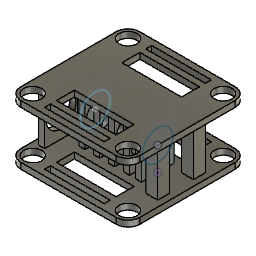
ROV frame sketch v1 (Autodesk Fusion 360 design; units mm, degrees)
Autodesk Fusion 360 part; units mm, degrees
sketch "Sketch3" plane through (0, 0, 0) normal (0, 0, 1) x (1, 0, 0)
  line L0 (80, 100) -> (-80, 100)
  line L1 (-100, 80) -> (-100, -80)
  line L2 (-80, -100) -> (80, -100)
  line L3 (100, -80) -> (100, 80)
  line L4 (100, 100) -> (-94.1421, -94.1421) construction
  line L5 (-100, 100) -> (100, -100) construction
  circle A0 centre (80, -80) radius 15
  circle A1 centre (80, 80) radius 15
  circle A2 centre (-80, -80) radius 15
  line L6 (-90, -5) -> (-90, -60)
  line L7 (-90, -60) -> (-80, -60)
  line L8 (-80, -60) -> (-80, -5)
  line L9 (-80, 45.4617) -> (-80, 5)
  line L10 (-80, 5) -> (-80, 60)
  line L11 (-80, 60) -> (-90, 60)
  line L12 (-90, 60) -> (-90, 5)
  line L13 (-90, -5) -> (-80, -5)
  line L14 (-80, 5) -> (-90, 5)
  arc A3 (100, 80) -> (80, 100) centre (80, 80) ccw
  arc A4 (80, -100) -> (100, -80) centre (80, -80) ccw
  arc A5 (-100, -80) -> (-80, -100) centre (-80, -80) ccw
  arc A6 (-80, 100) -> (-100, 80) centre (-80, 80) ccw
  line L15 (-50, 90) -> (50, 90)
  line L16 (50, 90) -> (50, 80)
  line L17 (50, 80) -> (-50, 80)
  line L18 (-50, 80) -> (-50, 90)
  line L19 (-50, -80) -> (50, -80)
  line L20 (50, -80) -> (50, -90)
  line L21 (50, -90) -> (-50, -90)
  line L22 (-50, -90) -> (-50, -80)
  line L23 (-80, -5) -> (-80, -60)
  line L24 (-80, 5) -> (-80, 60)
  circle A7 centre (-80, 80) radius 15
  line L25 (70, -20) -> (90, -20)
  line L26 (90, -20) -> (90, -40)
  line L27 (90, -40) -> (70, -40)
  line L28 (70, -40) -> (70, -20)
  line L29 (70, 20) -> (90, 20)
  line L30 (90, 20) -> (90, 40)
  line L31 (90, 40) -> (70, 40)
  line L32 (70, 40) -> (70, 20)
  line L33 (-50, 70) -> (50, 70)
  line L34 (50, 70) -> (50, 40)
  line L35 (50, 40) -> (-50, 40)
  line L36 (-50, 40) -> (-50, 70)
  line L37 (50, -70) -> (-50, -70)
  line L38 (-50, -70) -> (-50, -40)
  line L39 (-50, -40) -> (50, -40)
  line L40 (50, -40) -> (50, -70)
  line L41 (-45, -27.5) -> (-55, -27.5)
  line L42 (-55, -27.5) -> (-55, 27.5)
  line L43 (-55, 27.5) -> (-45, 27.5)
  line L44 (-45, 27.5) -> (-45, -27.5)
  line L45 (-45, -27.5) -> (-55, 27.5) construction
  line L46 (-55, -27.5) -> (-45, 27.5) construction
  line L47 (-20, -27.5) -> (-30, -27.5)
  line L48 (-30, -27.5) -> (-30, 27.5)
  line L49 (-30, 27.5) -> (-20, 27.5)
  line L50 (-20, 27.5) -> (-20, -27.5)
  line L51 (-20, -27.5) -> (-30, 27.5) construction
  line L52 (-30, -27.5) -> (-20, 27.5) construction
  line L53 (-5, 27.5) -> (5, 27.5)
  line L54 (5, 27.5) -> (5, -27.5)
  line L55 (5, -27.5) -> (-5, -27.5)
  line L56 (-5, -27.5) -> (-5, 27.5)
  line L57 (30, 27.5) -> (20, 27.5)
  line L58 (20, 27.5) -> (20, -27.5)
  line L59 (20, -27.5) -> (30, -27.5)
  line L60 (30, -27.5) -> (30, 27.5)
  line L61 (21.1538, -21.1538) -> (20, -27.5) construction
  line L62 (20, 27.5) -> (21.1538, 21.1538) construction
  line L63 (50, 27.5) -> (40, 27.5)
  line L64 (40, 27.5) -> (40, -27.5)
  line L65 (40, -27.5) -> (50, -27.5)
  line L66 (50, -27.5) -> (50, 27.5)
  point P0 (-50, 0)
  point P1 (-25, 0)
  point P2 (25, 0)
  point P3 (45, 0)
  dimension "d5" = 30
  dimension "d7" = 30
  dimension "d10" = 30
  dimension "d17" = 55
  dimension "d19" = 55
  dimension "d23" = 30
  dimension "d31" = 10
  dimension "d32" = 55
  dimension "d33" = 10
  dimension "d34" = 55
  dimension "d35" = 10
  dimension "d36" = 55
  dimension "d38" = 10
  dimension "d39" = 55
  dimension "d40" = 20
  dimension "d41" = 10
  dimension "d42" = 55
  constraint horizontal L0
  constraint perpendicular L0 L1
  constraint parallel L0 L2
  constraint parallel L1 L3
  constraint vertical L6
  constraint horizontal L7
  constraint vertical L8
  constraint vertical L9
  constraint vertical L10
  constraint horizontal L11
  constraint vertical L12
  constraint horizontal L13
  constraint horizontal L14
  constraint coincident A1.centre A3.centre
  constraint coincident A0.centre A4.centre
  constraint coincident A2.centre A5.centre
  constraint horizontal L15
  constraint vertical L16
  constraint horizontal L17
  constraint vertical L18
  constraint horizontal L19
  constraint vertical L20
  constraint horizontal L21
  constraint vertical L22
  constraint coincident A5 L4.end
  constraint concentric A6 A7
  constraint horizontal L25
  constraint vertical L26
  constraint horizontal L27
  constraint vertical L28
  constraint horizontal L29
  constraint vertical L30
  constraint horizontal L31
  constraint vertical L32
  constraint horizontal L33
  constraint vertical L34
  constraint horizontal L35
  constraint vertical L36
  constraint horizontal L37
  constraint vertical L38
  constraint horizontal L39
  constraint vertical L40
  constraint horizontal L41
  constraint perpendicular L41 L42
  constraint parallel L41 L43
  constraint parallel L42 L44
  constraint coincident L45 P0
  constraint coincident L46 P0
  constraint horizontal L47
  constraint perpendicular L47 L48
  constraint parallel L47 L49
  constraint parallel L48 L50
  constraint coincident L51 P1
  constraint coincident L52 P1
  constraint horizontal L53
  constraint perpendicular L53 L54
  constraint parallel L53 L55
  constraint parallel L54 L56
  constraint horizontal L57
  constraint perpendicular L57 L58
  constraint parallel L57 L59
  constraint parallel L58 L60
  constraint coincident L61 P2
  constraint coincident L62 P2
  constraint horizontal L63
  constraint perpendicular L63 L64
  constraint parallel L63 L65
  constraint parallel L64 L66
  constraint coincident L5 L61.start
  constraint coincident L4 L62.end
  measures "d5" diameter of A0
  measures "d7" diameter of A1
  measures "d10" diameter of A2
  measures "d17" distance of L6.end L6.start
  measures "d19" distance of L11.end L12.end
  measures "d23" diameter of A7
  measures "d31" distance of L42.end L43.end
  measures "d32" distance of L41.end L42.end
  measures "d33" distance of L48.end L49.end
  measures "d34" distance of L47.end L48.end
  measures "d35" distance of L54.end L55.end
  measures "d36" distance of L53.end L54.end
  measures "d38" distance of L58.end L59.end
  measures "d39" distance of L57.end L58.end
  measures "d40" distance of P2 P3
  measures "d41" distance of L64.end L65.end
  measures "d42" distance of L63.end L64.end
  measures "d52" diameter of L5.start
extrude "Extrude2" add sketch "Sketch3" against normal blind 10 contours L0 L1 L2 L3 A3 A4 A5 A6 | L6 L7 L8 L13 L23 | L9 L10 L11 L12 L14 L24 | L25 L26 L27 L28 | L29 L30 L31 L32 | L41 L42 L43 L44 | L47 L48 L49 L50 | L53 L54 L55 L56 | L57 L58 L59 L60 | L63 L64 L65 L66
extrude "Extrude3" add sketch "Sketch3" along normal blind 80 contours L6 L7 L8 L13 L23 | L9 L10 L11 L12 L14 L24
extrude "Extrude4" add sketch "Sketch3" along normal blind 80 contours L41 L42 L43 L44 | L47 L48 L49 L50 | L53 L54 L55 L56 | L57 L58 L59 L60 | L63 L64 L65 L66
sketch "Sketch5" plane through (50, 0, 0) normal (1, 0, 0) x (0, 1, 0)
  line L0 (-27.5, 0) -> (27.5, 0)
  line L1 (27.5, 0) -> (27.5, 80)
  line L2 (27.5, 80) -> (-27.5, 80)
  line L3 (-27.5, 80) -> (-27.5, 0)
  circle A0 centre (0, 40) radius 25
  line L4 (-27.5, 40) -> (-25, 40)
  line L5 (25, 40) -> (27.5, 40)
  dimension "d45" = 40
  dimension "d46" = 50
  constraint midpoint L3 L4.start
  constraint coincident A0 L4.end
  constraint perpendicular L3 L4
  constraint coincident A0 L5.start
  constraint midpoint L1 L5.end
  constraint perpendicular L1 L5
  measures "d45" distance of origin A0.centre
  measures "d46" diameter of A0
extrude "Extrude5" cut sketch "Sketch5" against normal blind 105 contours A0
extrude "Extrude6" cut sketch "Sketch5" against normal blind 105 contours L1 L2 L3 A0 L4 L5
sketch "Sketch6" plane through (-80, 0, 0) normal (1, 0, 0) x (0, 1, 0)
  line L0 (5, 0) -> (60, 0)
  line L1 (60, 0) -> (60, 80)
  line L2 (60, 80) -> (5, 80)
  line L3 (5, 80) -> (5, 0)
  circle A0 centre (32.5, 40) radius 25
  dimension "d52" = 50
  measures "d52" diameter of A0
sketch "Sketch7" plane through (-80, 0, 0) normal (1, 0, 0) x (0, 1, 0)
  line L0 (-60, 0) -> (-5, 0)
  line L1 (-5, 0) -> (-5, 80)
  line L2 (-5, 80) -> (-60, 80)
  line L3 (-60, 80) -> (-60, 0)
  circle A0 centre (-32.5, 40) radius 25
  dimension "d54" = 50
  measures "d54" diameter of A0
extrude "Extrude7" cut sketch "Sketch6" sketch "Sketch7" against normal blind 10 contours A0 of sketch 2 contours A0
ref_plane "WorkPlane1" through (0, 0, 80) normal (0, 0, 1) x (1, 0, 0)
sketch "Sketch8" plane through (0, 0, 80) normal (0, 0, 1) x (1, 0, 0)
  circle A0 centre (80, -80) radius 15
  circle A1 centre (-80, -80) radius 15
  circle A2 centre (80, 80) radius 15
  circle A3 centre (-80, 80) radius 15
  line L0 (40.0189, 27.5) -> (50.0189, 27.5)
  line L1 (50.0189, 27.5) -> (50.0189, -27.5)
  line L2 (50.0189, -27.5) -> (40.0189, -27.5)
  line L3 (40.0189, -27.5) -> (40.0189, 27.5)
  line L4 (40.0189, 27.5) -> (50.0189, -27.5) construction
  line L5 (50.0189, 27.5) -> (40.0189, -27.5) construction
  line L6 (20.082, 27.5) -> (30.082, 27.5)
  line L7 (30.082, 27.5) -> (30.082, -27.5)
  line L8 (30.082, -27.5) -> (20.082, -27.5)
  line L9 (20.082, -27.5) -> (20.082, 27.5)
  line L10 (20.082, 27.5) -> (30.082, -27.5) construction
  line L11 (30.082, 27.5) -> (20.082, -27.5) construction
  line L12 (-5, 27.5) -> (5, 27.5)
  line L13 (5, 27.5) -> (5, -27.5)
  line L14 (5, -27.5) -> (-5, -27.5)
  line L15 (-5, -27.5) -> (-5, 27.5)
  line L16 (-5, 27.5) -> (5, -27.5) construction
  line L17 (5, 27.5) -> (-5, -27.5) construction
  line L18 (-29.7604, 27.5) -> (-19.7604, 27.5)
  line L19 (-19.7604, 27.5) -> (-19.7604, -27.5)
  line L20 (-19.7604, -27.5) -> (-29.7604, -27.5)
  line L21 (-29.7604, -27.5) -> (-29.7604, 27.5)
  line L22 (-29.7604, 27.5) -> (-19.7604, -27.5) construction
  line L23 (-19.7604, 27.5) -> (-29.7604, -27.5) construction
  line L24 (-55, 27.5) -> (-45, 27.5)
  line L25 (-45, 27.5) -> (-45, -27.5)
  line L26 (-45, -27.5) -> (-55, -27.5)
  line L27 (-55, -27.5) -> (-55, 27.5)
  line L28 (-55, 27.5) -> (-45, -27.5) construction
  line L29 (-45, 27.5) -> (-55, -27.5) construction
  line L30 (50, -90) -> (-50, -90)
  line L31 (-50, -90) -> (-50, -80)
  line L32 (-50, -80) -> (50, -80)
  line L33 (50, -80) -> (50, -90)
  line L34 (50, -70) -> (-50, -70)
  line L35 (-50, -70) -> (-50, -40)
  line L36 (-50, -40) -> (50, -40)
  line L37 (50, -40) -> (50, -70)
  line L38 (50, 40) -> (-50, 40)
  line L39 (-50, 40) -> (-50, 70)
  line L40 (-50, 70) -> (50, 70)
  line L41 (50, 70) -> (50, 40)
  line L42 (50, 80) -> (-50, 80)
  line L43 (-50, 80) -> (-50, 90)
  line L44 (-50, 90) -> (50, 90)
  line L45 (50, 90) -> (50, 80)
  line L46 (80, -100) -> (-80, -100)
  line L47 (-100, -80) -> (-100, 80)
  line L48 (-80, 100) -> (80, 100)
  line L49 (100, 80) -> (100, -80)
  arc A4 (80, -100) -> (100, -80) centre (80, -80) ccw
  arc A5 (-100, -80) -> (-80, -100) centre (-80, -80) ccw
  arc A6 (-80, 100) -> (-100, 80) centre (-80, 80) ccw
  arc A7 (100, 80) -> (80, 100) centre (80, 80) ccw
  point P0 (45.0189, 0)
  point P1 (25.082, 0)
  point P2 (-24.7604, 0)
  point P3 (-50, 0)
  dimension "d58" = 30
  dimension "d59" = 30
  dimension "d60" = 30
  dimension "d61" = 30
  dimension "d62" = 10
  dimension "d63" = 55
  dimension "d64" = 10
  dimension "d65" = 55
  dimension "d66" = 10
  dimension "d67" = 55
  dimension "d68" = 10
  dimension "d69" = 55
  dimension "d70" = 10
  dimension "d71" = 55
  constraint horizontal L0
  constraint perpendicular L0 L1
  constraint parallel L0 L2
  constraint parallel L1 L3
  constraint coincident L4 P0
  constraint coincident L5 P0
  constraint horizontal L6
  constraint perpendicular L6 L7
  constraint parallel L6 L8
  constraint parallel L7 L9
  constraint coincident L10 P1
  constraint coincident L11 P1
  constraint horizontal L12
  constraint perpendicular L12 L13
  constraint parallel L12 L14
  constraint parallel L13 L15
  constraint coincident L16 origin
  constraint coincident L17 origin
  constraint horizontal L18
  constraint perpendicular L18 L19
  constraint parallel L18 L20
  constraint parallel L19 L21
  constraint coincident L22 P2
  constraint coincident L23 P2
  constraint horizontal L24
  constraint perpendicular L24 L25
  constraint parallel L24 L26
  constraint parallel L25 L27
  constraint coincident L28 P3
  constraint coincident L29 P3
  constraint horizontal L30
  constraint vertical L31
  constraint horizontal L32
  constraint vertical L33
  constraint horizontal L34
  constraint vertical L35
  constraint horizontal L36
  constraint vertical L37
  constraint horizontal L38
  constraint vertical L39
  constraint horizontal L40
  constraint vertical L41
  constraint horizontal L42
  constraint vertical L43
  constraint horizontal L44
  constraint vertical L45
  constraint horizontal L46
  constraint vertical L47
  constraint horizontal L48
  constraint vertical L49
  constraint coincident A0.centre A4.centre
  constraint coincident A1.centre A5.centre
  constraint coincident A3.centre A6.centre
  constraint coincident A2.centre A7.centre
  measures "d58" diameter of A0
  measures "d59" diameter of A1
  measures "d60" diameter of A2
  measures "d61" diameter of A3
  measures "d62" distance of L1.end L2.end
  measures "d63" distance of L0.end L1.end
  measures "d64" distance of L7.end L8.end
  measures "d65" distance of L6.end L7.end
  measures "d66" distance of L13.end L14.end
  measures "d67" distance of L12.end L13.end
  measures "d68" distance of L19.end L20.end
  measures "d69" distance of L18.end L19.end
  measures "d70" distance of L25.end L26.end
  measures "d71" distance of L24.end L25.end
extrude "Extrude8" add sketch "Sketch8" along normal blind 10
extrude "Extrude9" add sketch "Sketch3" along normal blind 80 contours L25 L26 L27 L28 | L29 L30 L31 L32
extrude "Extrude10" add sketch "Sketch8" along normal blind 10 and the other way blind 40 contours L0 L1 L2 L3 | L6 L7 L8 L9 | L12 L13 L14 L15 | L18 L19 L20 L21 | L24 L25 L26 L27
extrude "Extrude11" cut sketch "Sketch5" against normal blind 120 contours A0
sketch "Sketch9" plane through (50, 0, 40) normal (1, 0, 0) x (0, 1, 0)
  circle A0 centre (0, 0) radius 25
  dimension "d82" = 50
  constraint coincident A0.centre origin
  measures "d82" diameter of A0
sketch "Sketch10" plane through (-55, 0, 0) normal (-1, 0, 0) x (0, -1, 0)
  circle A0 centre (0, 40) radius 25
  line L0 (-27.5, 80) -> (-27.5, 0)
  line L1 (-27.5, 0) -> (27.5, 0)
  line L2 (27.5, 0) -> (27.5, 80)
  line L3 (27.5, 80) -> (-27.5, 80)
  circle A1 centre (0, 40) radius 25
  constraint concentric A0 A1
sketch "Sketch11" plane through (50.0189, 0, 0) normal (1, 0, 0) x (0, 1, 0)
  line L0 (27.5, 80) -> (-27.5, 80)
  line L1 (-27.5, 80) -> (-27.5, 40)
  line L2 (-27.5, 40) -> (27.5, 40)
  line L3 (27.5, 40) -> (27.5, 80)
  circle A0 centre (0, 40) radius 25
  dimension "d83" = 50
  constraint midpoint L2 A0.centre
  measures "d83" diameter of A0
extrude "Extrude12" cut sketch "Sketch11" against normal blind 10 contours L2 A0 picked at (0.7158, 49.5521)
